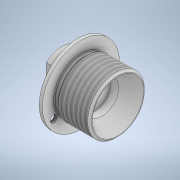
# Autodesk Inventor part: Чертеж 2
Saved by Autodesk Inventor 2020 (Build 240168000, 168)
## iProperties
Created: 2020-04-16
Part Number: Чертеж 2
Material: Типовые
Document SubType Name: Modeling
Designer: User
Density: 1 g/cm^3
Appearance: По умолчанию
Mass: 196.083 g
Surface Area: 362.427 cm^2
Volume: 196.083 cm^3
Author: User
Autodesk Inventor part; units mm, degrees
ref_plane "YZ Plane" through (0, 0, 0) normal (1, 0, 0) x (0, 1, 0)
ref_plane "XZ Plane" through (0, 0, 0) normal (0, 1, 0) x (-1, 0, 0)
ref_plane "XY Plane" through (0, 0, 0) normal (0, 0, 1) x (1, 0, 0)
sketch "Эскиз1" plane through (0, 0, 0) normal (0, 0, 1) x (1, 0, 0)
  line L0 (0, 0) -> (0, 30)
  line L1 (0, 30) -> (20, 30)
  line L2 (20, 30) -> (20, 49)
  line L3 (20, 49) -> (24, 49)
  line L4 (24, 49) -> (24, 33.8)
  line L5 (24, 33.8) -> (29.2, 33.8)
  line L6 (29.2, 33.8) -> (31.4, 36)
  line L7 (31.4, 36) -> (71, 36)
  line L8 (71, 36) -> (71, 0)
  line L9 (71, 0) -> (0, 0)
  dimension "d0" = 60
  dimension "d1" = 98
  dimension "d2" = 4
  dimension "d3" = 20
  dimension "d5" = 72
  dimension "d6" = 45
  dimension "d7" = 5.2
  dimension "d8" = 47
  dimension "d9" = 67.6
  constraints: 20 end point, 6 perpendicular, 2 vertical, 1 parallel
  measures "d0" diameter of L1 L9
  measures "d1" diameter of L3 L9
  measures "d2" distance of L2.end L3.end
  measures "d3" distance of L0.end L1.end
  measures "d5" diameter of L7 L9
  measures "d6" angle of L7 L6
  measures "d7" distance of L4.end L5.end
  measures "d8" distance between parallel lines of L4 L8
  measures "d9" diameter of L5 L9
revolve "Вращение1" add sketch "Эскиз1" angle 360 about axis through (71, 0, 0) along (-1, 0, 0)
sketch "Эскиз2" plane through (0, 0, 0) normal (0, 1, 0) x (-1, 0, 0)
  point P0 (0, 0)
sketch "Эскиз3" plane through (0, 0, 0) normal (0, 1, 0) x (-1, 0, 0)
  line L0 (0, -30) -> (0, 30) projected
  line L1 (-20, -30) -> (-20, 30) projected
  line L2 (-20, -49) -> (-20, 49) projected
  line L3 (-24, -49) -> (-24, 49) projected
  line L4 (-24, -33.8) -> (-24, 33.8) projected
  line L5 (-29.2, -33.8) -> (-29.2, 33.8) projected
  line L6 (-31.4, -36) -> (-31.4, 36) projected
  line L7 (-71, -36) -> (-71, 36) projected
  line L8 (0, -30) -> (-15, -30)
  line L9 (-15, -30) -> (-15, -20)
  line L10 (-15, -20) -> (0, -20)
  line L11 (0, -20) -> (0, -30)
  line L12 (0, -30) -> (0, 30) projected
  line L13 (0, 20) -> (-15, 20)
  line L14 (-15, 20) -> (-15, 30)
  line L15 (-15, 30) -> (0, 30)
  line L16 (0, 30) -> (0, 20)
  line L17 (-20, -30) -> (0, -30) projected
  line L18 (-20, 30) -> (0, 30) projected
  point P0 (0, 0)
  point P1 (0, -20)
  dimension "d11" = 40
  dimension "d12" = 15
  constraints: 16 end point, 4 parallel, 4 point on line, 2 equal length, 2 horizontal, 2 perpendicular
  measures "d11" distance between parallel lines of L13 L10
  measures "d12" distance from line of L14 L15.end
extrude "Выдавливание1" cut sketch "Эскиз3" against normal through all both and the other way through all contours L8 L9 L10 L0 | L13 L14 L15 L0
sketch "Эскиз4" plane through (0, 0, 0) normal (0, 1, 0) x (-1, 0, 0)
  line L0 (-15, -20) -> (0, -20) projected
  line L1 (0, 20) -> (0, -20) projected
  line L2 (0, 20) -> (-15, 20) projected
  line L3 (-15, 20) -> (-15, 20) projected
  line L4 (-15, 20) -> (0, 20) projected
  line L5 (0, -20) -> (0, 20) projected
  line L6 (0, -20) -> (-15, -20) projected
  line L7 (-15, -20) -> (-15, -20) projected
  line L8 (-20, -30) -> (-20, 30) projected
  line L9 (-15, -20) -> (0, -20) projected
  line L10 (14.2, 0) -> (-85.2, 0) projected
  circle A0 centre (-11, 0) radius 7
  point P0 (0, 0)
  dimension "d15" = 14
  dimension "d46" = 11
  constraints: 1 centre point, 1 point on line
  measures "d15" diameter of A0
  measures "d46" distance from line of L1 A0.centre
extrude "Выдавливание2" cut sketch "Эскиз4" along normal through all both and the other way through all
sketch "Эскиз5" plane through (0, 0, 0) normal (1, 0, 0) x (0, 1, 0)
  circle A0 centre (0, 0) radius 30 projected
  circle A1 centre (0, 0) radius 49 projected
  line L0 (0, -68.6) -> (0, 68.6) projected
  circle A2 centre (-20, 34.641) radius 4.5
  line L1 (0, 0) -> (0, 86.4455)
  line L2 (0, 0) -> (-51.3565, 88.952)
  line L3 (0, 0) -> (50.4363, 29.1194)
  line L4 (-71.9154, 0) -> (71.9969, 0) projected
  point P0 (0, 0)
  dimension "d20" = 30
  dimension "d21" = 9
  dimension "d22" = 30
  dimension "d23" = 40
  constraints: 6 end point, 2 point on line, 1 centre point
  measures "d20" angle of L2 L1
  measures "d21" diameter of A2
  measures "d22" angle of L4 L3
  measures "d23" distance from line of A2.centre L3
sketch "Эскиз6" plane through (0, 0, 0) normal (1, 0, 0) x (0, 1, 0)
  point P0 (0, 0)
extrude "Выдавливание3" cut sketch "Эскиз5" along normal blind 24 contours L2 A2 | A2 L2
thread "Резьба1" size "M72x6" class "6g" standard "ANSI Metric M Profile" full length
fillet "Сопряжение1" radius 1 1 edges at (29.2, -33.8, 0)
fillet "Сопряжение2" radius 1 1 edges at (24, -33.8, 0)
chamfer "Фаска2" distance 2.5 angle 45 1 edges at (71, -36, 0) measured on face at (71, -35.5, 0)
sketch "Эскиз7" plane through (71, 0, 0) normal (1, 0, 0) x (0, 0, -1)
  point P0 (0, 0)
hole "Отверстие1" at (71, 0, 0) direction (-1, 0, 0) diameter 42 depth 30
chamfer "Фаска3" distance 20 angle 30 1 edges at (71, 0, 21) measured on face at (70.5, 0, 21)
